Autodesk Fusion 360 part; units mm, degrees
(part 2 of 3)
sketch "Sketch5" plane through (0, 0, 1.5) normal (0, 0, 1) x (-1, 0, 0)
  line L0 (17.5, -111.5) -> (17.5, -101.5)
  line L1 (17.5, -101.5) -> (28.75, -101.5)
  line L2 (28.75, -101.5) -> (28.75, -111.5)
  line L3 (28.75, -111.5) -> (17.5, -111.5)
  arc A0 (29, -9) -> (20, 0) centre (20, -9) ccw
  line L4 (20, 0) -> (-20, 0)
  arc A1 (-20, 0) -> (-29, -9) centre (-20, -9) ccw
  line L5 (-29, -9) -> (-29, -117)
  arc A2 (-29, -117) -> (-20, -126) centre (-20, -117) ccw
  line L6 (-20, -126) -> (20, -126)
  arc A3 (20, -126) -> (29, -117) centre (20, -117) ccw
  line L7 (29, -117) -> (29, -9)
  circle A4 centre (-23.5, -110) radius 1.5
  line L8 (-23.5, -108.5) -> (-27.7, -108.5)
  line L9 (-27.7, -108.5) -> (-27.7, -83)
  line L10 (-27.7, -83) -> (-22.7, -83)
  line L11 (-22.7, -83) -> (-22.7, -108.5)
  line L12 (-22.7, -108.5) -> (-23.5, -108.5)
  circle A5 centre (23.5, -24) radius 1.5
  circle A6 centre (23.5, -116) radius 1.5
  circle A7 centre (-23.5, -30) radius 1.5
  line L13 (-22.7, -58.9) -> (-27.7, -58.9)
  line L14 (-27.7, -58.9) -> (-27.7, -33.4)
  line L15 (-27.7, -33.4) -> (-22.7, -33.4)
  line L16 (-22.7, -33.4) -> (-22.7, -58.9)
  line L17 (27.7, -98) -> (22.7, -98)
  line L18 (22.7, -98) -> (22.7, -77.5)
  line L19 (22.7, -77.5) -> (27.7, -77.5)
  line L20 (27.7, -77.5) -> (27.7, -98)
  line L21 (-22.7, -81.7) -> (-27.7, -81.7)
  line L22 (-27.7, -81.7) -> (-27.7, -61.2)
  line L23 (-27.7, -61.2) -> (-22.7, -61.2)
  line L24 (-22.7, -61.2) -> (-22.7, -81.7)
  line L25 (27.7, -52.4) -> (22.7, -52.4)
  line L26 (22.7, -52.4) -> (22.7, -26.9)
  line L27 (22.7, -26.9) -> (27.7, -26.9)
  line L28 (27.7, -26.9) -> (27.7, -52.4)
  line L29 (27.7, -75.2) -> (22.7, -75.2)
  line L30 (22.7, -75.2) -> (22.7, -54.7)
  line L31 (22.7, -54.7) -> (27.7, -54.7)
  line L32 (27.7, -54.7) -> (27.7, -75.2)
  line L33 (-29, -126) -> (-11, -126)
  line L34 (-11, -126) -> (-18.5, -126)
  line L35 (-11, -126) -> (-11, -127.2)
  line L36 (-11, -127.2) -> (-18.5, -127.2)
  line L37 (-18.5, -127.2) -> (-18.5, -126)
  line L38 (-11, -126) -> (-11, -122)
  line L39 (-11, -122) -> (-18.5, -122)
  line L40 (-18.5, -122) -> (-18.5, -126)
  line L41 (-11, -125) -> (-7.5, -125)
  line L42 (-7.5, -125.5) -> (-7.5, -127.8)
  line L43 (-7.5, -125.5) -> (-5.5, -125.5)
  line L44 (-5.5, -125.5) -> (-5.5, -127.8)
  line L45 (-5.5, -127.8) -> (-7.5, -127.8)
  line L46 (-5.5, -126.65) -> (-5, -126.65) construction
  line L47 (-3, -127.8) -> (-5, -127.8)
  line L48 (-3, -125.5) -> (-3, -127.8)
  line L49 (-5, -125.5) -> (-3, -125.5)
  line L50 (-5, -125.5) -> (-5, -127.8)
  line L51 (-0.5, -127.8) -> (-2.5, -127.8)
  line L52 (-0.5, -125.5) -> (-0.5, -127.8)
  line L53 (-2.5, -125.5) -> (-0.5, -125.5)
  line L54 (-2.5, -125.5) -> (-2.5, -127.8)
  line L55 (2, -127.8) -> (0, -127.8)
  line L56 (0, -125.5) -> (0, -127.8)
  line L57 (2, -125.5) -> (2, -127.8)
  line L58 (0, -125.5) -> (2, -125.5)
  line L59 (2, -127.8) -> (0, -127.8)
  line L60 (2, -125.5) -> (2, -127.8)
  line L61 (0, -125.5) -> (2, -125.5)
  line L62 (0, -125.5) -> (0, -127.8)
  line L63 (-0.5, -125.5) -> (-0.5, -127.8)
  line L64 (-0.5, -127.8) -> (-2.5, -127.8)
  line L65 (-2.5, -125.5) -> (-2.5, -127.8)
  line L66 (-2.5, -125.5) -> (-0.5, -125.5)
  line L67 (-5, -125.5) -> (-3, -125.5)
  line L68 (-3, -125.5) -> (-3, -127.8)
  line L69 (-3, -127.8) -> (-5, -127.8)
  line L70 (-5, -125.5) -> (-5, -127.8)
  line L71 (-5.5, -127.8) -> (-7.5, -127.8)
  line L72 (-5.5, -125.5) -> (-5.5, -127.8)
  line L73 (-7.5, -125.5) -> (-5.5, -125.5)
  line L74 (-7.5, -125.5) -> (-7.5, -127.8)
  line L75 (14.5, -125.5) -> (14.5, -127.8)
  line L76 (14.5, -127.8) -> (12.5, -127.8)
  line L77 (12.5, -125.5) -> (14.5, -125.5)
  line L78 (12.5, -125.5) -> (12.5, -127.8)
  line L79 (12, -125.5) -> (12, -127.8)
  line L80 (12, -127.8) -> (10, -127.8)
  line L81 (10, -125.5) -> (10, -127.8)
  line L82 (10, -125.5) -> (12, -125.5)
  line L83 (9.5, -127.8) -> (7.5, -127.8)
  line L84 (9.5, -125.5) -> (9.5, -127.8)
  line L85 (7.5, -125.5) -> (9.5, -125.5)
  line L86 (7.5, -125.5) -> (7.5, -127.8)
  line L87 (7, -125.5) -> (7, -127.8)
  line L88 (7, -127.8) -> (5, -127.8)
  line L89 (5, -125.5) -> (7, -125.5)
  line L90 (5, -125.5) -> (5, -127.8)
  line L91 (-29, -9) -> (-20.7, -9)
  line L92 (-20.7, -0.0273) -> (-20.7, -7.1273)
  line L93 (-20.7, -7.1273) -> (-13.2, -7.1273)
  line L94 (-13.2, -7.1273) -> (-13.2, 0)
  line L95 (-20.7, -0.0273) -> (-13.2, 0)
  line L96 (-16.95, -0.0136) -> (-16.9558, 1.5864)
  line L97 (-16.95, -0.0136) -> (-16.9573, 1.9864)
  arc A8 (-13.2, 0) -> (-20.7, -0.0273) centre (-16.9369, -3.6082) ccw
  circle A9 centre (-16.9409, -2.5136) radius 4.5
  dimension "d100" = 18
  dimension "d101" = 7.5
  dimension "d102" = 1.2
  dimension "d103" = 4
  dimension "d112" = 3.5
  dimension "d114" = 2.3
  dimension "d115" = 2
  dimension "d116" = 2.3
  dimension "d117" = 0.5
  dimension "d118" = 2.3
  dimension "d119" = 2
  dimension "d120" = 2.3
  dimension "d121" = 2.3
  dimension "d122" = 2
  dimension "d123" = 2.3
  dimension "d124" = 2.3
  dimension "d125" = 2
  dimension "d126" = 2.3
  dimension "d143" = 2.3
  dimension "d144" = 2
  dimension "d145" = 2.3
  dimension "d146" = 2.3
  dimension "d147" = 2
  dimension "d148" = 2.3
  dimension "d149" = 2.3
  dimension "d150" = 2
  dimension "d151" = 2.3
  dimension "d152" = 2.3
  dimension "d153" = 2
  dimension "d154" = 2.3
  dimension "d155" = 2.3
  dimension "d156" = 2
  dimension "d157" = 2.3
  dimension "d158" = 2.3
  dimension "d159" = 2
  dimension "d160" = 2.3
  dimension "d161" = 2.3
  dimension "d162" = 2
  dimension "d163" = 2.3
  dimension "d164" = 2.3
  dimension "d165" = 2
  dimension "d166" = 2.3
  dimension "d169" = 8.3
  dimension "d170" = 7.1
  dimension "d171" = 7.5
  dimension "d172" = 1.6
  dimension "d173" = 2
  dimension "d174" = 9
  constraint perpendicular L5 L33
  constraint parallel L33 L34
  constraint perpendicular L6 L35
  constraint perpendicular L35 L36
  constraint perpendicular L34 L38
  constraint perpendicular L38 L39
  constraint coincident L38 L41.start
  constraint perpendicular L38 L41
  constraint perpendicular L6 L42
  constraint perpendicular L42 L43
  constraint perpendicular L6 L44
  constraint midpoint L44 L46.start
  constraint perpendicular L44 L46
  constraint perpendicular L49 L50
  constraint perpendicular L53 L54
  constraint perpendicular L56 L58
  constraint perpendicular L73 L74
  constraint perpendicular L67 L70
  constraint perpendicular L65 L66
  constraint perpendicular L61 L62
  constraint perpendicular L89 L90
  constraint perpendicular L85 L86
  constraint perpendicular L81 L82
  constraint perpendicular L77 L78
  constraint coincident A1.end L5.start
  constraint perpendicular L5 L91
  constraint coincident A1 L92.start
  constraint perpendicular L91 L92
  constraint perpendicular L92 L93
  constraint coincident L4 L94.end
  constraint perpendicular L4 L94
  constraint midpoint L95 L96.start
  constraint perpendicular L95 L96
  constraint perpendicular L95 L97
  constraint coincident L96.end A8
  constraint coincident L97.end A9
  measures "d100" distance of L33.start L33.end
  measures "d101" distance of L33.end L34.end
  measures "d102" distance of L33.end L35.end
  measures "d103" distance of L33.end L38.end
  measures "d112" distance of L41.start L41.end
  measures "d114" distance of L42.start L42.end
  measures "d115" distance of L42.start L43.end
  measures "d116" distance of L43.end L44.end
  measures "d117" distance of L46.start L46.end
  measures "d118" distance of L49.start L47.end
  measures "d119" distance of L49.start L48.start
  measures "d120" distance of L47.start L48.start
  measures "d121" distance of L53.start L51.end
  measures "d122" distance of L53.start L52.start
  measures "d123" distance of L51.start L52.start
  measures "d124" distance of L55.end L56.start
  measures "d125" distance of L57.start L56.start
  measures "d126" distance of L57.start L55.start
  measures "d143" distance of L42.start L42.end
  measures "d144" distance of L42.start L43.end
  measures "d145" distance of L44.end L43.end
  measures "d146" distance of L49.start L47.end
  measures "d147" distance of L49.start L48.start
  measures "d148" distance of L47.start L48.start
  measures "d149" distance of L51.end L53.start
  measures "d150" distance of L52.start L53.start
  measures "d151" distance of L52.start L51.start
  measures "d152" distance of L55.end L56.start
  measures "d153" distance of L57.start L56.start
  measures "d154" distance of L57.start L55.start
  measures "d155" distance of L89.start L88.end
  measures "d156" distance of L89.start L87.start
  measures "d157" distance of L87.end L87.start
  measures "d158" distance of L85.start L83.end
  measures "d159" distance of L85.start L84.start
  measures "d160" distance of L83.start L84.start
  measures "d161" distance of L80.end L81.start
  measures "d162" distance of L79.start L81.start
  measures "d163" distance of L79.start L79.end
  measures "d164" distance of L76.end L77.start
  measures "d165" distance of L75.start L77.start
  measures "d166" distance of L75.start L75.end
  measures "d169" distance of A1.end L91.end
  measures "d170" distance of L92.start L92.end
  measures "d171" distance of L92.end L93.end
  measures "d172" distance of L96.start L96.end
  measures "d173" distance of L96.start L97.end
  measures "d174" diameter of A9
extrude "Extrude8" add sketch "Sketch5" along normal blind 3 separate body contours L6 L33 L34 L38 L39 L40 | L6 L33 L34 L35 L36 L37 makes body 2
fillet "Fillet2" radius 1 6 edges at (18.5, 124, 1.5) (18.5, 126.6, 1.5) (18.5, 124, 4.5) (18.5, 126.6, 4.5) (11, 124.6, 4.5) (11, 124.6, 1.5) on bodies 2
sketch "Sketch6" plane through (0, 127.2, 0) normal (0, 1, 0) x (-1, 0, 0)
  arc A0 (-12, 1.5) -> (-11, 2.5) centre (-12, 2.5) ccw
  line L0 (-11, 2.5) -> (-11, 3.5)
  arc A1 (-11, 3.5) -> (-12, 4.5) centre (-12, 3.5) ccw
  line L1 (-12, 4.5) -> (-17.5, 4.5)
  arc A2 (-17.5, 4.5) -> (-18.5, 3.5) centre (-17.5, 3.5) ccw
  line L2 (-18.5, 3.5) -> (-18.5, 2.5)
  arc A3 (-18.5, 2.5) -> (-17.5, 1.5) centre (-17.5, 2.5) ccw
  line L3 (-17.5, 1.5) -> (-12, 1.5)
  line L4 (-17, 2) -> (-12.5, 2)
  arc A4 (-12.5, 2) -> (-12.5, 4) centre (-12.5, 3) ccw
  line L5 (-12.5, 4) -> (-17, 4)
  arc A5 (-17, 4) -> (-17, 2) centre (-17, 3) ccw
  line L6 (-17, 3) -> (-12.5, 3) construction
  constraint tangent L4 A4
  constraint tangent A4 L5
  constraint parallel L4 L5
  constraint tangent L5 A5
  constraint tangent L4 A5
  constraint perpendicular L0 L6
extrude "Extrude9" cut sketch "Sketch6" against normal blind 5 contours L4 A4 L5 A5 bodies 2
sketch "Sketch7" plane through (0, 122.2, 0) normal (0, 1, 0) x (-1, 0, 0)
  arc A0 (-17, 4) -> (-17, 2) centre (-17, 3) ccw
  line L0 (-17, 2) -> (-12.5, 2)
  arc A1 (-12.5, 2) -> (-12.5, 4) centre (-12.5, 3) ccw
  line L1 (-12.5, 4) -> (-17, 4)
  line L2 (-17, 3) -> (-12.5, 3)
  line L3 (-12.5, 3) -> (-12.5, 2.5)
  line L4 (-12.5, 2.5) -> (-17, 2.5)
  line L5 (-17, 2.5) -> (-17, 3)
  constraint horizontal L2
  constraint vertical L3
  constraint horizontal L4
  constraint vertical L5
  constraint coincident A0.centre L2.start
extrude "Extrude10" add sketch "Sketch7" along normal blind 4 contours L2 L3 L4 L5 bodies 2
extrude "Extrude11" add sketch "Sketch5" along normal blind 2.3 contours L6 L55 L56 L57 L59 L60 L62 | L6 L56 L57 L58 L60 L61 L62 | L6 L42 L43 L44 L72 L73 L74 | L6 L42 L44 L45 L71 L72 L74 | L6 L51 L52 L54 L63 L64 L65 | L6 L52 L53 L54 L63 L65 L66 | L6 L48 L49 L50 L67 L68 L70 | L6 L47 L48 L50 L68 L69 L70 bodies 1
ref_plane "WorkPlane1" through (-1, 126.65, 2.65) normal (1, 0, 0) x (0, 1, 0)
sketch "Sketch8" plane through (-1, 0, 0) normal (1, 0, 0) x (0, 1, 0)
  line L0 (123.5, 1.5) -> (123.5, 2.1)
  line L1 (124.05, 2.65) -> (125.5, 2.65)
  arc A0 (124.05, 2.65) -> (123.5, 2.1) centre (124.05, 2.1) ccw
  line L2 (127.8, 2.65) -> (133.8, 2.65)
  dimension "d132" = 0.55
  dimension "d137" = 6
  constraint tangent L0 A0
  constraint tangent L1 A0
  constraint parallel L1 L2
  measures "d132" radius of A0
  measures "d137" distance of L2.start L2.end
pipe "Pipe1" add square section size 0.5 path "Sketch8" along L1 A0 L0 separate body makes body 3
copy_body "CopyPasteBodies1" bodies 3 makes body 4
move_body "Move1" bodies 4 to x (1, 0, 0) y (0, 1, 0) z (0, 0, 1) at (2.5, 0, 0)
copy_body "CopyPasteBodies2" bodies 4 makes body 5
move_body "Move2" bodies 5 to x (1, 0, 0) y (0, 1, 0) z (0, 0, 1) at (2.5, 0, 0)
copy_body "CopyPasteBodies3" bodies 5 makes body 6
move_body "Move3" bodies 6 to x (1, 0, 0) y (0, 1, 0) z (0, 0, 1) at (2.5, 0, 0)
pipe "Pipe2" add square section size 0.5 path "Sketch8" along L2 separate body makes body 7
copy_body "CopyPasteBodies4" bodies 7 makes body 8
move_body "Move4" bodies 8 to x (1, 0, 0) y (0, 1, 0) z (0, 0, 1) at (2.5, 0, 0)
copy_body "CopyPasteBodies5" bodies 8 makes body 9
move_body "Move5" bodies 9 to x (1, 0, 0) y (0, 1, 0) z (0, 0, 1) at (2.5, 0, 0)
copy_body "CopyPasteBodies6" bodies 9 makes body 10
move_body "Move6" bodies 10 to x (1, 0, 0) y (0, 1, 0) z (0, 0, 1) at (2.5, 0, 0)
chamfer "Chamfer1" distance 0.15 angle 45 16 edges at (-1, 133.8, 2.9) (-0.75, 133.8, 2.65) (-1, 133.8, 2.4) (-1.25, 133.8, 2.65) (6.5, 133.8, 2.9) (6.75, 133.8, 2.65) (6.25, 133.8, 2.65) (6.5, 133.8, 2.4) (1.5, 133.8, 2.9) (1.75, 133.8, 2.65) (1.25, 133.8, 2.65) (1.5, 133.8, 2.4) (4, 133.8, 2.9) (4.25, 133.8, 2.65) (3.75, 133.8, 2.65) (4, 133.8, 2.4) on bodies 7 8 9 10
extrude "Extrude12" add sketch "Sketch5" along normal blind 2.3 contours L6 L75 L76 L78 | L6 L75 L77 L78 | L6 L79 L80 L81 | L6 L79 L81 L82 | L6 L83 L84 L86 | L6 L84 L85 L86 | L6 L87 L88 L90 | L6 L87 L89 L90 bodies 1
copy_body "CopyPasteBodies7" bodies 3 7 9 6 8 10 4 5 makes body 11 makes body 12 makes body 13 makes body 14 makes body 15 makes body 16 makes body 17 makes body 18
move_body "Move7" bodies 11 12 13 14 15 16 17 18 to x (1, 0, 0) y (0, 1, 0) z (0, 0, 1) at (-12.5, 0, 0)
extrude "Extrude13" add sketch "Sketch5" along normal blind 2 separate body contours L92 L94 L95 A9 | L4 L96 L97 A8 A9 | L4 A1 L96 L97 A8 A9 | L92 L93 L94 A9 makes body 19 at (14.7234, -1.0912, 2.8333) makes body 20 at (16.95, 3.3386, 1.5)
extrude "Extrude14" add sketch "Sketch5" along normal blind 3.8 and the other way blind -2.3 separate body contours L4 L95 L96 L97 | L92 L94 L95 A9 | L4 L96 L97 A8 A9 | L94 A9 | L97 A8 A9 | L4 A1 L95 L96 L97 | L4 A1 L96 L97 A8 A9 | L97 A8 A9 | L92 A9 makes body 21
sketch "Sketch9" plane through (0, 0, 0) normal (0, 0, -1) x (1, 0, 0)
  circle A0 centre (23.5, -110) radius 1.5
  arc A1 (-20, 0) -> (-29, -9) centre (-20, -9) ccw
  line L0 (-29, -9) -> (-29, -117)
  arc A2 (-29, -117) -> (-20, -126) centre (-20, -117) ccw
  line L1 (-20, -126) -> (20, -126)
  arc A3 (20, -126) -> (29, -117) centre (20, -117) ccw
  line L2 (29, -117) -> (29, -9)
  arc A4 (29, -9) -> (20, 0) centre (20, -9) ccw
  line L3 (20, 0) -> (-20, 0)
  circle A5 centre (-23.5, -24) radius 1.5
  circle A6 centre (-23.5, -116) radius 1.5
  circle A7 centre (23.5, -30) radius 1.5
  circle A8 centre (-20, -9) radius 3.85
  circle A9 centre (20, -9) radius 3.85
  circle A10 centre (-15, -105) radius 3.85
  circle A11 centre (15, -105) radius 3.85
  circle A12 centre (-20, -9) radius 3.25
  circle A13 centre (20, -9) radius 3.25
  circle A14 centre (-15, -105) radius 3.25
  circle A15 centre (15, -105) radius 3.25
  dimension "d181" = 7.7
  dimension "d182" = 7.7
  dimension "d183" = 7.7
  dimension "d184" = 7.7
  dimension "d185" = 6.5
  dimension "d186" = 6.5
  dimension "d187" = 6.5
  dimension "d188" = 6.5
  constraint concentric A1 A8
  constraint concentric A4 A9
  constraint concentric A8 A12
  constraint concentric A4 A13
  constraint concentric A10 A14
  constraint concentric A11 A15
  measures "d181" diameter of A8
  measures "d182" diameter of A9
  measures "d183" diameter of A10
  measures "d184" diameter of A11
  measures "d185" diameter of A12
  measures "d186" diameter of A13
  measures "d187" diameter of A14
  measures "d188" diameter of A15
extrude "Extrude15" add sketch "Sketch9" along normal blind 5.4 contours A12 | A13 | A14 | A15 bodies 1
extrude "Extrude16" add sketch "Sketch9" along normal blind 1 contours A8 | A9 | A10 | A11 bodies 1
equation "d62 = 7.2 mm + 1.5 mm"

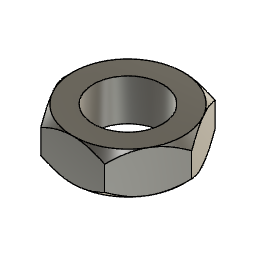
design "5mm Nut"
Autodesk Fusion 360 part; units mm, degrees
sketch "Sketch1" plane through (0, 0, 0) normal (0, 0, 1) x (1, 0, 0)
  circle A0 centre (0, 0) radius 2.5
  circle A1 centre (0, 0) radius 4
  line L0 (-2.3094, 4) -> (-4.6188, 0)
  line L1 (-4.6188, 0) -> (-2.3094, -4)
  line L2 (-2.3094, -4) -> (2.3094, -4)
  line L3 (2.3094, -4) -> (4.6188, 0)
  line L4 (4.6188, 0) -> (2.3094, 4)
  line L5 (2.3094, 4) -> (-2.3094, 4)
  dimension "d1" = 5
  dimension "d2" = 8
  constraint coincident A0.centre A1.centre
  measures "d1" diameter of A0
  measures "d2" diameter of A1
extrude "Extrude1" add sketch "Sketch1" along normal blind 3
sketch "Sketch2" plane through (0, 0, 3) normal (0, 0, 1) x (-1, 0, 0)
  circle A0 centre (0, 0) radius 2.5
  line L0 (-2.3094, -4) -> (2.3094, -4)
  line L1 (2.3094, -4) -> (4.6188, 0)
  line L2 (4.6188, 0) -> (2.3094, 4)
  line L3 (2.3094, 4) -> (-2.3094, 4)
  line L4 (-2.3094, 4) -> (-4.6188, 0)
  line L5 (-4.6188, 0) -> (-2.3094, -4)
  circle A1 centre (0, 0) radius 4
  constraint coincident A0.centre A1.centre
  constraint tangent L0 A1
extrude "Extrude2" cut sketch "Sketch2" against normal blind 6 draft 45 contours A1 keep common part
sketch "Sketch3" plane through (0, 0, 0) normal (0, 0, -1) x (1, 0, 0)
  circle A0 centre (0, 0) radius 2.5
  line L0 (-2.3094, -4) -> (2.3094, -4)
  line L1 (2.3094, -4) -> (4.6188, 0)
  line L2 (4.6188, 0) -> (2.3094, 4)
  line L3 (2.3094, 4) -> (-2.3094, 4)
  line L4 (-2.3094, 4) -> (-4.6188, 0)
  line L5 (-4.6188, 0) -> (-2.3094, -4)
  circle A1 centre (0, 0) radius 4
  constraint concentric A0 A1
  constraint tangent L3 A1
extrude "Extrude3" cut sketch "Sketch3" against normal blind 9 draft 45 contours A1 keep common part

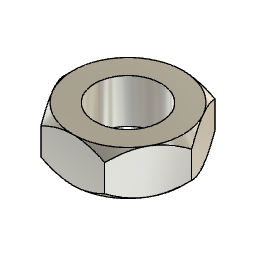
design "3mm_Nut"
Autodesk Fusion 360 part; units mm, degrees
sketch "Sketch1" plane through (0, 0, 0) normal (0, 0, 1) x (1, 0, 0)
  circle A0 centre (0, 0) radius 1.5
  line L0 (-1.4434, 2.5) -> (-2.8868, 0)
  line L1 (-2.8868, 0) -> (-1.4434, -2.5)
  line L2 (-1.4434, -2.5) -> (1.4434, -2.5)
  line L3 (1.4434, -2.5) -> (2.8868, 0)
  line L4 (2.8868, 0) -> (1.4434, 2.5)
  line L5 (1.4434, 2.5) -> (-1.4434, 2.5)
  dimension "d1" = 3
  constraint coincident A0.centre origin
  measures "d1" diameter of A0
extrude "Extrude1" add sketch "Sketch1" along normal blind 2
sketch "Sketch2" plane through (0, 0, 2) normal (0, 0, 1) x (-1, 0, 0)
  circle A0 centre (0, 0) radius 1.5
  line L0 (-1.4434, -2.5) -> (1.4434, -2.5)
  line L1 (1.4434, -2.5) -> (2.8868, 0)
  line L2 (2.8868, 0) -> (1.4434, 2.5)
  line L3 (1.4434, 2.5) -> (-1.4434, 2.5)
  line L4 (-1.4434, 2.5) -> (-2.8868, 0)
  line L5 (-2.8868, 0) -> (-1.4434, -2.5)
  circle A1 centre (0, 0) radius 2.5
  constraint coincident A0.centre A1.centre
  constraint tangent L0 A1
extrude "Extrude2" cut sketch "Sketch2" against normal blind 7 draft 45 contours A1 keep common part
sketch "Sketch3" plane through (0, 0, 0) normal (0, 0, -1) x (1, 0, 0)
  circle A0 centre (0, 0) radius 1.5
  line L0 (-1.4434, -2.5) -> (1.4434, -2.5)
  line L1 (1.4434, -2.5) -> (2.8868, 0)
  line L2 (2.8868, 0) -> (1.4434, 2.5)
  line L3 (1.4434, 2.5) -> (-1.4434, 2.5)
  line L4 (-1.4434, 2.5) -> (-2.8868, 0)
  line L5 (-2.8868, 0) -> (-1.4434, -2.5)
  circle A1 centre (0, 0) radius 2.5
  constraint concentric A0 A1
  constraint tangent L0 A1
extrude "Extrude3" cut sketch "Sketch3" against normal blind 5 draft 45 contours A1 keep common part

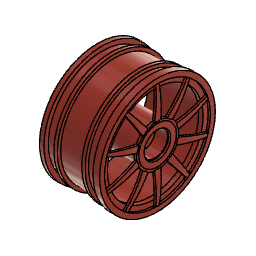
design "Wheel2"
Autodesk Fusion 360 part; units mm, degrees
sketch "Sketch1" plane through (0, 0, 0) normal (0, 1, 0) x (1, 0, 0)
  line L0 (0, -26) -> (-2, -26)
  line L1 (-2, -26) -> (-2, -24)
  line L2 (-2, -24) -> (-6, -24)
  line L3 (-6, -24) -> (-6, -25.5)
  line L4 (-6, -25.5) -> (-7.5, -25.5)
  line L5 (-7.5, -25.5) -> (-7.5, -24)
  line L6 (-7.5, -24) -> (-18.5, -24)
  line L7 (-13, -24) -> (-13, -27.5) construction
  line L8 (-18.5, -25.5) -> (-18.5, -24)
  line L9 (-20, -25.5) -> (-18.5, -25.5)
  line L10 (-20, -24) -> (-20, -25.5)
  line L11 (-24, -24) -> (-20, -24)
  line L12 (-24, -26) -> (-24, -24)
  line L13 (-26, -26) -> (-24, -26)
  line L14 (-13, -24) -> (-13, -27.5) construction
  line L15 (-26, -26) -> (-26, -13)
  line L16 (0, -26) -> (0, -13)
  line L17 (-33, -13) -> (4.5762, -13) construction
  line L18 (0, 0) -> (0, -13)
  line L19 (0, 0) -> (-2, 0)
  line L20 (-2, 0) -> (-2, -2)
  line L21 (-2, -2) -> (-6, -2)
  line L22 (-6, -2) -> (-6, -0.5)
  line L23 (-6, -0.5) -> (-7.5, -0.5)
  line L24 (-7.5, -0.5) -> (-7.5, -2)
  line L25 (-7.5, -2) -> (-18.5, -2)
  line L26 (-18.5, -0.5) -> (-18.5, -2)
  line L27 (-20, -0.5) -> (-18.5, -0.5)
  line L28 (-20, -2) -> (-20, -0.5)
  line L29 (-24, -2) -> (-20, -2)
  line L30 (-24, 0) -> (-24, -2)
  line L31 (-26, 0) -> (-24, 0)
  line L32 (-26, 0) -> (-26, -13)
  line L33 (-26, 0) -> (-26, -3)
  line L34 (-26, -3) -> (-2, -3)
  line L35 (-2, -3) -> (-2, -4.5)
  line L36 (-2, -4.5) -> (0, -4.5)
  dimension "d2" = 26
  dimension "d3" = 2
  dimension "d4" = 2
  dimension "d5" = 4
  dimension "d6" = 1.5
  dimension "d7" = 1.5
  dimension "d8" = 1.5
  dimension "d9" = 11
  dimension "d10" = 13
  dimension "d11" = 13
  dimension "d12" = 3
  dimension "d13" = 1.5
  constraint perpendicular L0 L1
  constraint perpendicular L1 L2
  constraint perpendicular L2 L3
  constraint perpendicular L3 L4
  constraint perpendicular L4 L5
  constraint perpendicular L5 L6
  constraint midpoint L6 L7.start
  constraint perpendicular L6 L7
  constraint symmetric L0.start L7 L13.start
  constraint symmetric L0.end L7 L12.start
  constraint symmetric L1.end L7 L11.start
  constraint symmetric L2.end L7 L10.start
  constraint symmetric L3.end L7 L9.start
  constraint symmetric L4.end L7 L8.start
  constraint symmetric L5.end L7 L6.end
  constraint symmetric L14.start L7 L7.start
  constraint symmetric L14.end L7 L7.end
  constraint perpendicular L13 L15
  constraint perpendicular L0 L16
  constraint perpendicular L16 L17
  constraint symmetric L0.start L17 L18.start
  constraint symmetric L0.end L17 L19.end
  constraint symmetric L1.end L17 L20.end
  constraint symmetric L2.end L17 L21.end
  constraint symmetric L3.end L17 L22.end
  constraint symmetric L4.end L17 L23.end
  constraint symmetric L5.end L17 L24.end
  constraint symmetric L6.end L17 L25.end
  constraint symmetric L8.start L17 L26.start
  constraint symmetric L9.start L17 L27.start
  constraint symmetric L10.start L17 L28.start
  constraint symmetric L11.start L17 L29.start
  constraint symmetric L12.start L17 L30.start
  constraint symmetric L13.start L17 L31.start
  constraint symmetric L15.end L17 L32.end
  constraint symmetric L16.end L17 L18.end
  constraint perpendicular L31 L33
  constraint perpendicular L33 L34
  constraint perpendicular L34 L35
  constraint coincident L18 L36.end
  constraint perpendicular L18 L36
  measures "d2" distance of L18.start L0.start
  measures "d3" distance of L0.start L0.end
  measures "d4" distance of L0.end L1.end
  measures "d5" distance of L1.end L2.end
  measures "d6" distance of L2.end L3.end
  measures "d7" distance of L3.end L4.end
  measures "d8" distance of L4.end L5.end
  measures "d9" distance of L5.end L6.end
  measures "d10" distance of L13.start L15.end
  measures "d11" distance of L0.start L16.end
  measures "d12" distance of L31.start L33.end
  measures "d13" distance of L34.end L35.end
revolve "Revolve1" add sketch "Sketch1" angle 360 about axis through (0, 0, 26) along (-1, 0, 0) contours L18 L19 L20 L21 L22 L23 L24 L25 L26 L27 L28 L29 L30 L31 L32 L33 L34 L35 L36 makes body 1
ref_plane "WorkPlane1" through (0, 0, 26) normal (1, 0, 0) x (0, 0, -1)
sketch "Sketch2" plane through (0, 0, 0) normal (1, 0, 0) x (0, 1, 0)
  circle A0 centre (0, 26) radius 21.5
  circle A1 centre (0, 26) radius 5.5
  circle A2 centre (0, 26) radius 8.5
  circle A3 centre (0, 26) radius 6
  dimension "d16" = 11
  dimension "d17" = 17
  dimension "d18" = 12
  constraint concentric A0 A1
  constraint concentric A0 A2
  constraint concentric A2 A3
  measures "d16" diameter of A1
  measures "d17" diameter of A2
  measures "d18" diameter of A3
extrude "Extrude1" add sketch "Sketch2" along normal blind 1 separate body contours A2 makes body 2
sketch "Sketch3" plane through (0, 0, 0) normal (1, 0, 0) x (0, 1, 0)
  circle A0 centre (0, 26) radius 26
  circle A1 centre (0, 26) radius 21.5
  circle A2 centre (0, 26) radius 23.75
  dimension "d21" = 47.5
  constraint concentric A0 A2
  measures "d21" diameter of A2
extrude "Extrude2" add sketch "Sketch3" along normal blind 1 contours A0 bodies 1
extrude "Extrude3" add sketch "Sketch2" against normal blind 5.5 separate body contours A3 makes body 3
extrude "Extrude4" add sketch "Sketch2" against normal blind 16 contours A2 bodies 2 3
extrude "Extrude5" add sketch "Sketch2" along normal blind -6 and the other way blind 5.5 separate body contours A1 makes body 4
sketch "Sketch4" plane through (0, 0, 0) normal (1, 0, 0) x (0, 1, 0)
  circle A0 centre (0, 26) radius 1.5
  dimension "d32" = 3
  measures "d32" diameter of A0
extrude "Extrude6" cut sketch "Sketch4" against normal blind 30 bodies 4
sketch "Sketch5" plane through (-6, 0, 0) normal (-1, 0, 0) x (0, -1, 0)
  circle A0 centre (0, 26) radius 1.5
  circle A1 centre (0, 26) radius 5.5
  line L0 (-3.4641, 32) -> (-6.9282, 26)
  line L1 (-6.9282, 26) -> (-3.4641, 20)
  line L2 (-3.4641, 20) -> (3.4641, 20)
  line L3 (3.4641, 20) -> (6.9282, 26)
  line L4 (6.9282, 26) -> (3.4641, 32)
  line L5 (3.4641, 32) -> (-3.4641, 32)
  point P0 (0, 26)
  dimension "d35" = 12
  constraint coincident P0 A0.centre
  measures "d35" vertical distance of L0.start L2.end
extrude "Extrude7" cut sketch "Sketch5" along normal blind 47 contours L0 L1 L2 L3 L4 L5 bodies 2
ref_plane "WorkPlane3" through (-2.2433, 0, 26) normal (0, -1, 0) x (0, 0, 1)
sketch "Sketch6" plane through (0, 0, 0) normal (0, -1, 0) x (-1, 0, 0)
  arc A0 (-1, -34.5) -> (-1, -49.75) centre (55, -42.125) ccw
  arc A1 (-0.0254, -34.4777) -> (-0.0556, -49.7496) centre (55.4716, -42.2236) ccw
  line L0 (-1, -34.5) -> (-0.9617, -34.2189)
  line L1 (-0.9617, -34.2189) -> (0.0019, -34.3501)
  line L2 (-0.0254, -34.4777) -> (0.0019, -34.3501)
  line L3 (-0.0556, -49.7496) -> (-1, -49.75)
  constraint tangent A0 A1
  constraint tangent A0 L0
  constraint perpendicular L0 L1
extrude "Extrude8" add sketch "Sketch6" along normal blind 1.5 and the other way blind 1.5 bodies 1 4 2
ref_plane "WorkPlane4" through (1.5167, 0.4718, 42.125) normal (1, 0, 0) x (0, 0, -1)
sketch "Sketch7" plane through (1.5167, 0, 0) normal (1, 0, 0) x (0, 1, 0)
  line L0 (1.5, 49.75) -> (0.0073, 49.75)
  arc A0 (0.0073, 49.75) -> (-0.0073, 49.75) centre (0, 26) ccw
  line L1 (-0.0073, 49.75) -> (-1.5, 49.75)
  line L2 (-1.5, 49.75) -> (-1.5, 34.5)
  line L3 (-1.5, 34.5) -> (0, 34.5)
  line L4 (0, 34.5) -> (1.5, 34.5)
  line L5 (1.5, 34.5) -> (1.5, 49.75)
  line L6 (-0.7536, 49.75) -> (-1.5, 34.365)
  line L7 (-1.5, 34.365) -> (0, 34.5)
  line L8 (0, 34.5) -> (1.4987, 34.365)
  line L9 (1.4987, 34.365) -> (0.7536, 49.75)
  line L10 (0.7536, 49.75) -> (-0.7536, 49.75)
  constraint midpoint L1 L6.start
  constraint coincident L3.end L4.start
  constraint midpoint L0 L9.end
extrude "Extrude9" cut sketch "Sketch7" against normal blind 1.5 contours L0 L4 L5 L9 | L1 L2 L3 L6 bodies 1
pattern_circular "C-Pattern1" count 10 over 360 about axis through (1, 0, 26) along (1, 0, 0) of "Extrude8", "Extrude9"
sketch "Sketch8" plane through (1, 0, 0) normal (1, 0, 0) x (0, 1, 0)
  circle A0 centre (0, 26) radius 6
  arc A1 (0, 34.5) -> (-4.9962, 32.8766) centre (0, 26) ccw
  arc A2 (-4.9962, 32.8766) -> (-8.084, 28.6266) centre (0, 26) ccw
  arc A3 (-8.084, 28.6266) -> (-8.084, 23.3734) centre (0, 26) ccw
  arc A4 (-8.084, 23.3734) -> (-4.9962, 19.1234) centre (0, 26) ccw
  arc A5 (-4.9962, 19.1234) -> (0, 17.5) centre (0, 26) ccw
  arc A6 (0, 17.5) -> (4.9962, 19.1234) centre (0, 26) ccw
  arc A7 (4.9962, 19.1234) -> (8.084, 23.3734) centre (0, 26) ccw
  arc A8 (8.084, 23.3734) -> (8.084, 28.6266) centre (0, 26) ccw
  arc A9 (8.084, 28.6266) -> (4.9962, 32.8766) centre (0, 26) ccw
  arc A10 (4.9962, 32.8766) -> (0, 34.5) centre (0, 26) ccw
  circle A11 centre (0, 26) radius 9.5
  dimension "d49" = 19
  constraint concentric A0 A11
  measures "d49" diameter of A11
extrude "Extrude10" add sketch "Sketch8" along normal blind -1 and the other way blind -0.1 contours A11 bodies 1

design "Pixy2"
Autodesk Fusion 360 part; units mm, degrees
sketch "Sketch1" plane through (0, 0, 0) normal (1, 0, 0) x (0, 1, 0)
  line L0 (0, 0) -> (0, 47.7) construction
  line L1 (-8.85, 0) -> (8.85, 0)
  line L2 (-8.85, 0) -> (-8.85, 4.5)
  line L3 (8.85, 0) -> (8.85, 4.5)
  line L4 (10.85, 6.5) -> (18.85, 6.5)
  line L5 (-10.85, 6.5) -> (-18.85, 6.5)
  line L6 (-18.85, 6.5) -> (-18.85, 42)
  line L7 (18.85, 6.5) -> (18.85, 42)
  line L8 (-18.85, 42) -> (-8.85, 42)
  line L9 (-8.85, 42) -> (-8.85, 43.8)
  line L10 (18.85, 42) -> (8.85, 42)
  line L11 (8.85, 42) -> (8.85, 43.8)
  line L12 (-2.5, 47.7) -> (2.5, 47.7)
  line L13 (-8.85, 43.8) -> (-2.5, 47.7)
  line L14 (8.85, 43.8) -> (2.5, 47.7)
  line L15 (-8.85, 4.5) -> (-10.85, 6.5)
  line L16 (8.85, 4.5) -> (10.85, 6.5)
  point P0 (-8.85, 6.5)
  point P1 (8.85, 6.5)
  dimension "d1" = 47.7
  dimension "d2" = 17.7
  dimension "d5" = 10
  dimension "d6" = 10
  dimension "d7" = 35.5
  dimension "d8" = 35.5
  dimension "d9" = 10
  dimension "d10" = 1.8
  dimension "d11" = 10
  dimension "d12" = 1.8
  dimension "d13" = 5
  dimension "d15" = 2
  dimension "d16" = 2
  dimension "d17" = 2
  dimension "d18" = 2
  constraint coincident L0.start origin
  constraint vertical L0
  constraint horizontal L1
  constraint midpoint L0.start L1
  constraint perpendicular L1 L2
  constraint perpendicular L1 L3
  constraint perpendicular L3 L4
  constraint perpendicular L2 L5
  constraint perpendicular L5 L6
  constraint perpendicular L4 L7
  constraint perpendicular L6 L8
  constraint perpendicular L8 L9
  constraint perpendicular L7 L10
  constraint perpendicular L10 L11
  constraint horizontal L12
  constraint midpoint L0.end L12
  constraint coincident P0 L2
  constraint coincident P0 L5
  constraint coincident P1 L3
  constraint coincident P1 L4
  measures "d1" distance of L0.start L0.end
  measures "d2" distance of L1.start L1.end
  measures "d5" distance of P1 L4.end
  measures "d6" distance of P0 L5.end
  measures "d7" distance of L5.end L6.end
  measures "d8" distance of L4.end L7.end
  measures "d9" distance of L6.end L8.end
  measures "d10" distance of L8.end L9.end
  measures "d11" distance of L7.end L10.end
  measures "d12" distance of L10.end L11.end
  measures "d13" distance of L12.start L12.end
  measures "d15" distance of P0 L2.end
  measures "d16" distance of P0 L5.start
  measures "d17" distance of P1 L3.end
  measures "d18" distance of P1 L4.start
extrude "Extrude1" add sketch "Sketch1" along normal blind 1.5
sketch "Sketch2" plane through (0, 0, 0) normal (-1, 0, 0) x (0, -1, 0)
  line L0 (-8.85, 0) -> (8.85, 0)
  line L1 (8.85, 0) -> (8.85, 4.5)
  line L2 (8.85, 4.5) -> (10.85, 6.5)
  line L3 (10.85, 6.5) -> (18.85, 6.5)
  line L4 (18.85, 6.5) -> (18.85, 42)
  line L5 (18.85, 42) -> (8.85, 42)
  line L6 (8.85, 42) -> (8.85, 43.8)
  line L7 (8.85, 43.8) -> (2.5, 47.7)
  line L8 (2.5, 47.7) -> (-2.5, 47.7)
  line L9 (-2.5, 47.7) -> (-8.85, 43.8)
  line L10 (-8.85, 43.8) -> (-8.85, 42)
  line L11 (-8.85, 42) -> (-18.85, 42)
  line L12 (-18.85, 42) -> (-18.85, 6.5)
  line L13 (-18.85, 6.5) -> (-10.85, 6.5)
  line L14 (-10.85, 6.5) -> (-8.85, 4.5)
  line L15 (-8.85, 4.5) -> (-8.85, 0)
  line L16 (8.85, 43.8) -> (7.35, 43.8)
  line L17 (-8.85, 43.8) -> (-7.35, 43.8)
  line L18 (-7.35, 43.8) -> (7.35, 43.8)
  line L19 (-7.35, 43.8) -> (-7.35, 29.1)
  line L20 (8.1, 43.8) -> (8.1, 29.1)
  line L21 (-7.35, 29.1) -> (8.1, 29.1)
  line L22 (-2.15, 43.8) -> (2.15, 43.8)
  line L23 (-2.15, 43.8) -> (-2.15, 45.35)
  line L24 (2.15, 43.8) -> (2.15, 45.35)
  arc A0 (0, 47.5) -> (-2.15, 45.35) centre (0, 45.35) ccw
  arc A1 (2.15, 45.35) -> (0, 47.5) centre (0, 45.35) ccw
  line L25 (-25.85, 36.45) -> (11.15, 36.45) construction
  line L26 (-25.85, 36.45) -> (11.15, 36.45) construction
  arc A2 (0, 25.4) -> (2.15, 27.55) centre (0, 27.55) ccw
  line L27 (-2.15, 29.1) -> (-2.15, 27.55)
  arc A3 (-2.15, 27.55) -> (0, 25.4) centre (0, 27.55) ccw
  line L28 (2.15, 29.1) -> (2.15, 27.55)
  circle A4 centre (0, 45.35) radius 0.75
  circle A5 centre (0, 27.55) radius 0.75
  point P0 (-2.15, 47.5)
  point P1 (2.15, 47.5)
  dimension "d21" = 1.5
  dimension "d22" = 1.5
  dimension "d23" = 14.7
  dimension "d24" = 14.7
  dimension "d25" = 4.3
  dimension "d26" = 3.7
  dimension "d27" = 3.7
  dimension "d28" = 2.15
  dimension "d29" = 1.5
  dimension "d30" = 1.5
  constraint coincident L6.end L7.start
  constraint perpendicular L6 L16
  constraint coincident L9.end L10.start
  constraint perpendicular L10 L17
  constraint perpendicular L17 L19
  constraint midpoint L16 L20.start
  constraint perpendicular L16 L20
  constraint horizontal L22
  constraint midpoint L18 L22
  constraint perpendicular L22 L23
  constraint perpendicular L22 L24
  constraint coincident P0 L23
  constraint tangent L23 A0
  constraint coincident P1 L24
  constraint tangent L24 A1
  constraint equal A0 A1
  constraint coincident A0.start A1.end
  constraint horizontal L25
  constraint midpoint L19 L25
  constraint symmetric L22.start L25 L27.start
  constraint symmetric L22.end L25 L28.start
  constraint symmetric L23.end L25 L27.end
  constraint symmetric A0.start L25 A2.start
  constraint symmetric A0 L25 A3
  constraint symmetric L24.end L25 A2.end
  constraint symmetric A1 L25 A2
  constraint symmetric L26.start L25 L25.start
  constraint symmetric L26.end L25 L25.end
  constraint concentric A0 A4
  constraint concentric A3 A5
  measures "d21" distance of L6.end L16.end
  measures "d22" distance of L9.end L17.end
  measures "d23" distance of L17.end L19.end
  measures "d24" distance of L20.start L20.end
  measures "d25" distance of L22.start L22.end
  measures "d26" distance of L22.start P0
  measures "d27" distance of L22.end P1
  measures "d28" radius of A0
  measures "d29" diameter of A4
  measures "d30" diameter of A5
extrude "Extrude2" add sketch "Sketch2" along normal blind 4.2 contours L16 L18 L19 L20 L21 L22 | L18 L22 L23 L24 A0 A1 | L21 A2 L27 A3 L28
sketch "Sketch3" plane through (-4.2, 0, 0) normal (-1, 0, 0) x (0, -1, 0)
  circle A0 centre (0, 27.55) radius 0.75
  circle A1 centre (0, 45.35) radius 0.75
  line L0 (8.1, 43.8) -> (2.15, 43.8)
  line L1 (2.15, 43.8) -> (2.15, 45.35)
  arc A2 (2.15, 45.35) -> (-2.15, 45.35) centre (0, 45.35) ccw
  line L2 (-2.15, 45.35) -> (-2.15, 43.8)
  line L3 (-2.15, 43.8) -> (-7.35, 43.8)
  line L4 (-7.35, 43.8) -> (-7.35, 29.1)
  line L5 (-7.35, 29.1) -> (-2.15, 29.1)
  line L6 (-2.15, 29.1) -> (-2.15, 27.55)
  arc A3 (-2.15, 27.55) -> (2.15, 27.55) centre (0, 27.55) ccw
  line L7 (2.15, 27.55) -> (2.15, 29.1)
  line L8 (2.15, 29.1) -> (8.1, 29.1)
  line L9 (8.1, 29.1) -> (8.1, 43.8)
  line L10 (-7.35, 36.45) -> (8.1, 36.45) construction
  line L11 (0, 47.5) -> (0, 25.4) construction
  circle A4 centre (0, 36.45) radius 6.7
  dimension "d33" = 13.4
  constraint midpoint L4 L10.start
  constraint midpoint L9 L10.end
  constraint midpoint A2 L11.start
  constraint midpoint A3 L11.end
  constraint midpoint L11 A4.centre
  measures "d33" diameter of A4
extrude "Extrude3" add sketch "Sketch3" along normal blind 6.2 contours A4
sketch "Sketch4" plane through (0, -8.1, 0) normal (0, -1, 0) x (1, 0, 0)
  line L0 (0, 29.1) -> (0, 43.8)
  line L1 (0, 43.8) -> (-4.2, 43.8)
  line L2 (-4.2, 43.8) -> (-4.2, 29.1)
  line L3 (-4.2, 29.1) -> (0, 29.1)
  line L4 (-10.4, 43.15) -> (-10.4, 29.75)
  line L5 (-4.2, 29.75) -> (-4.2, 43.15)
  line L6 (-10.4, 43.15) -> (-6.7, 43.15)
  line L7 (-10.4, 29.75) -> (-6.7, 29.75)
  line L8 (-10.4, 43.15) -> (-5.4, 43.15)
  line L9 (-10.4, 29.75) -> (-5.4, 29.75)
  line L10 (-5.4, 43.15) -> (-5.4, 29.75)
  line L11 (-6.7, 43.15) -> (-6.7, 29.75)
  dimension "d36" = 3.7
  dimension "d37" = 3.7
  dimension "d38" = 5
  dimension "d39" = 5
  constraint coincident L4.start L6.start
  constraint perpendicular L4 L6
  constraint coincident L4.end L7.start
  constraint perpendicular L4 L7
  constraint perpendicular L4 L8
  constraint perpendicular L4 L9
  measures "d36" distance of L4.start L6.end
  measures "d37" distance of L4.end L7.end
  measures "d38" distance of L4.start L8.end
  measures "d39" distance of L4.end L9.end
ref_plane "WorkPlane1" through (-5.4, 0, 36.45) normal (-1, 0, 0) x (0, -1, 0)
sketch "Sketch5" plane through (-5.4, 0, 0) normal (-1, 0, 0) x (0, -1, 0)
  circle A0 centre (0, 36.45) radius 6.7
  circle A1 centre (0, 36.45) radius 6.7
  circle A2 centre (0, 36.45) radius 5.5
  dimension "d41" = 11
  constraint concentric A0 A1
  constraint concentric A1 A2
  measures "d41" diameter of A2
extrude "Extrude4" cut sketch "Sketch5" along normal blind 1.3
sketch "Sketch6" plane through (-10.4, 0, 0) normal (-1, 0, 0) x (0, -1, 0)
  circle A0 centre (0, 36.45) radius 6.7
  circle A1 centre (0, 36.45) radius 3.5
  circle A2 centre (0, 36.45) radius 1.25
  dimension "d44" = 7
  dimension "d45" = 2.5
  constraint concentric A0 A1
  constraint concentric A0 A2
  measures "d44" diameter of A1
  measures "d45" diameter of A2
extrude "Extrude5" add sketch "Sketch6" along normal blind 0.1 contours A1
sketch "Sketch7" plane through (1.5, 0, 0) normal (1, 0, 0) x (0, 1, 0)
  line L0 (-8.85, 0) -> (8.85, 0)
  line L1 (8.85, 0) -> (8.85, 4.5)
  line L2 (8.85, 4.5) -> (10.85, 6.5)
  line L3 (10.85, 6.5) -> (18.85, 6.5)
  line L4 (18.85, 6.5) -> (18.85, 42)
  line L5 (18.85, 42) -> (8.85, 42)
  line L6 (8.85, 42) -> (8.85, 43.8)
  line L7 (8.85, 43.8) -> (2.5, 47.7)
  line L8 (2.5, 47.7) -> (-2.5, 47.7)
  line L9 (-2.5, 47.7) -> (-8.85, 43.8)
  line L10 (-8.85, 43.8) -> (-8.85, 42)
  line L11 (-8.85, 42) -> (-18.85, 42)
  line L12 (-18.85, 42) -> (-18.85, 6.5)
  line L13 (-18.85, 6.5) -> (-10.85, 6.5)
  line L14 (-10.85, 6.5) -> (-8.85, 4.5)
  line L15 (-8.85, 4.5) -> (-8.85, 0)
  line L16 (-4.85, 0) -> (4.85, 0)
  line L17 (4.85, 0) -> (4.85, 3.5) construction
  line L18 (-4.85, 0) -> (-4.85, 3.5) construction
  circle A0 centre (-3.35, 3.5) radius 1.5
  circle A1 centre (3.35, 3.5) radius 1.5
  line L19 (15.35, 6.5) -> (15.35, 9) construction
  circle A2 centre (15.35, 10.5) radius 1.5
  line L20 (13.6, 13.4) -> (13.6, 20.9) construction
  line L21 (11.1, 13.4) -> (16.1, 13.4)
  line L22 (11.1, 13.4) -> (11.1, 20.9)
  line L23 (11.1, 20.9) -> (16.1, 20.9)
  line L24 (16.1, 20.9) -> (16.1, 13.4)
  line L25 (12.5002, 19.75) -> (11.9998, 19.75)
  line L26 (11.9998, 19.75) -> (11.9998, 20.25)
  line L27 (11.9998, 20.25) -> (12.5002, 20.25)
  line L28 (12.5002, 20.25) -> (12.5002, 19.75)
  line L29 (12.5002, 19.75) -> (11.9998, 20.25) construction
  line L30 (11.9998, 19.75) -> (12.5002, 20.25) construction
  line L31 (14.6998, 20.25) -> (15.2002, 20.25)
  line L32 (14.6998, 19.75) -> (14.6998, 20.25)
  line L33 (15.2002, 20.25) -> (15.2002, 19.75)
  line L34 (15.2002, 19.75) -> (14.6998, 19.75)
  line L35 (11.9998, 17.5) -> (12.5002, 17.5)
  line L36 (11.9998, 17) -> (11.9998, 17.5)
  line L37 (12.5002, 17.5) -> (12.5002, 17)
  line L38 (12.5002, 17) -> (11.9998, 17)
  line L39 (14.6998, 17.5) -> (15.2002, 17.5)
  line L40 (14.6998, 17) -> (14.6998, 17.5)
  line L41 (15.2002, 17.5) -> (15.2002, 17)
  line L42 (15.2002, 17) -> (14.6998, 17)
  line L43 (11.9998, 14.75) -> (12.5002, 14.75)
  line L44 (11.9998, 14.25) -> (11.9998, 14.75)
  line L45 (12.5002, 14.75) -> (12.5002, 14.25)
  line L46 (12.5002, 14.25) -> (11.9998, 14.25)
  line L47 (14.6998, 14.75) -> (15.2002, 14.75)
  line L48 (14.6998, 14.25) -> (14.6998, 14.75)
  line L49 (15.2002, 14.75) -> (15.2002, 14.25)
  line L50 (15.2002, 14.25) -> (14.6998, 14.25)
  point P0 (12.25, 20)
  dimension "d48" = 9.7
  dimension "d49" = 3.5
  dimension "d50" = 3.5
  dimension "d53" = 3
  dimension "d54" = 3
  dimension "d56" = 2.5
  dimension "d58" = 3
  dimension "d60" = 7.5
  dimension "d61" = 5
  dimension "d62" = 0.5
  dimension "d65" = 2.7
  dimension "d66" = -5.5
  constraint perpendicular L15 L16
  constraint midpoint L0 L16
  constraint perpendicular L0 L17
  constraint perpendicular L16 L18
  constraint coincident L18.end A0
  constraint coincident L17.end A1
  constraint coincident L3 L19.start
  constraint perpendicular L3 L19
  constraint coincident L19.end A2
  constraint horizontal L21
  constraint midpoint L20.start L21
  constraint perpendicular L21 L22
  constraint perpendicular L20 L23
  constraint perpendicular L21 L24
  constraint horizontal L25
  constraint perpendicular L25 L26
  constraint parallel L25 L27
  constraint parallel L26 L28
  constraint coincident L29 P0
  constraint coincident L30 P0
  measures "d48" distance of L16.start L16.end
  measures "d49" distance of L16.end L17.end
  measures "d50" distance of L16.start L18.end
  measures "d53" diameter of A0
  measures "d54" diameter of A1
  measures "d56" distance of L19.start L19.end
  measures "d58" diameter of A2
  measures "d60" distance of L20.start L20.end
  measures "d61" distance of L21.start L21.end
  measures "d62" distance of L25.end L26.end
extrude "Extrude6" add sketch "Sketch7" along normal blind 9 contours L25 L26 L27 L28 | L31 L32 L33 L34 | L35 L36 L37 L38 | L39 L40 L41 L42 | L43 L44 L45 L46 | L47 L48 L49 L50
extrude "Extrude7" add sketch "Sketch7" along normal blind 3 contours L21 L22 L23 L24
chamfer "Chamfer1" distance 0.2 angle 45 6 faces at (10.5, 12.3334, 19.9167) (10.5, 14.8666, 20.0833) (10.5, 14.8666, 17.3333) (10.5, 12.1666, 17.3333) (10.5, 12.1666, 14.5833) (10.5, 14.8666, 14.5833)
sketch "Sketch8" plane through (1.5, 0, 0) normal (1, 0, 0) x (0, 1, 0)
  line L0 (11.1, 13.4) -> (11.1, 20.9)
  line L1 (11.1, 20.9) -> (16.1, 20.9)
  line L2 (16.1, 20.9) -> (16.1, 13.4)
  line L3 (16.1, 13.4) -> (11.1, 13.4)
  line L4 (-8.85, 0) -> (8.85, 0)
  line L5 (8.85, 0) -> (8.85, 4.5)
  line L6 (8.85, 4.5) -> (10.85, 6.5)
  line L7 (10.85, 6.5) -> (18.85, 6.5)
  line L8 (18.85, 6.5) -> (18.85, 42)
  line L9 (18.85, 42) -> (8.85, 42)
  line L10 (8.85, 42) -> (8.85, 43.8)
  line L11 (8.85, 43.8) -> (2.5, 47.7)
  line L12 (2.5, 47.7) -> (-2.5, 47.7)
  line L13 (-2.5, 47.7) -> (-8.85, 43.8)
  line L14 (-8.85, 43.8) -> (-8.85, 42)
  line L15 (-8.85, 42) -> (-18.85, 42)
  line L16 (-18.85, 42) -> (-18.85, 6.5)
  line L17 (-18.85, 6.5) -> (-10.85, 6.5)
  line L18 (-10.85, 6.5) -> (-8.85, 4.5)
  line L19 (-8.85, 4.5) -> (-8.85, 0)
  line L20 (9.1614, 42) -> (18.1614, 42)
  line L21 (9.1614, 42) -> (9.1614, 22)
  line L22 (18.1614, 22) -> (9.1614, 22)
  line L23 (18.1614, 22) -> (18.1614, 42)
  line L24 (17.1614, 23) -> (17.1614, 41)
  line L25 (10.1614, 41) -> (17.1614, 41)
  line L26 (10.1614, 41) -> (10.1614, 23)
  line L27 (17.1614, 23) -> (10.1614, 23)
  line L28 (8.1614, 32) -> (10.1614, 32)
  line L29 (10.1614, 32) -> (10.1614, 34)
  line L30 (9.1614, 34) -> (10.1614, 34)
  line L31 (10.1614, 32) -> (10.1614, 30)
  line L32 (10.1614, 30) -> (9.1614, 30)
  line L33 (12, 38) -> (12.5, 38)
  line L34 (12.5, 38) -> (12.5, 37.5)
  line L35 (12.5, 37.5) -> (12, 37.5)
  line L36 (12, 37.5) -> (12, 38)
  line L37 (15, 38) -> (15.5, 38)
  line L38 (15, 37.5) -> (15, 38)
  line L39 (15.5, 38) -> (15.5, 37.5)
  line L40 (15.5, 37.5) -> (15, 37.5)
  line L41 (12, 35.25) -> (12.5, 35.25)
  line L42 (12, 34.75) -> (12, 35.25)
  line L43 (12.5, 35.25) -> (12.5, 34.75)
  line L44 (12.5, 34.75) -> (12, 34.75)
  line L45 (15, 35.25) -> (15.5, 35.25)
  line L46 (15, 34.75) -> (15, 35.25)
  line L47 (15.5, 35.25) -> (15.5, 34.75)
  line L48 (15.5, 34.75) -> (15, 34.75)
  line L49 (12, 32.5) -> (12.5, 32.5)
  line L50 (12, 32) -> (12, 32.5)
  line L51 (12.5, 32.5) -> (12.5, 32)
  line L52 (12.5, 32) -> (12, 32)
  line L53 (15, 32.5) -> (15.5, 32.5)
  line L54 (15, 32) -> (15, 32.5)
  line L55 (15.5, 32.5) -> (15.5, 32)
  line L56 (15.5, 32) -> (15, 32)
  line L57 (12, 29.75) -> (12.5, 29.75)
  line L58 (12, 29.25) -> (12, 29.75)
  line L59 (12.5, 29.75) -> (12.5, 29.25)
  line L60 (12.5, 29.25) -> (12, 29.25)
  line L61 (15, 29.75) -> (15.5, 29.75)
  line L62 (15, 29.25) -> (15, 29.75)
  line L63 (15.5, 29.75) -> (15.5, 29.25)
  line L64 (15.5, 29.25) -> (15, 29.25)
  line L65 (12, 27) -> (12.5, 27)
  line L66 (12, 26.5) -> (12, 27)
  line L67 (12.5, 27) -> (12.5, 26.5)
  line L68 (12.5, 26.5) -> (12, 26.5)
  line L69 (15, 27) -> (15.5, 27)
  line L70 (15, 26.5) -> (15, 27)
  line L71 (15.5, 27) -> (15.5, 26.5)
  line L72 (15.5, 26.5) -> (15, 26.5)
  dimension "d72" = 9
  dimension "d73" = 20
  dimension "d74" = 1
  dimension "d75" = 2
  dimension "d76" = 2
  dimension "d77" = 0.5
  dimension "d78" = 0.5
  dimension "d81" = 3
  dimension "d82" = -11
  constraint coincident L9 L20.start
  constraint perpendicular L9 L21
  constraint perpendicular L21 L22
  constraint perpendicular L9 L23
  constraint perpendicular L8 L28
  constraint midpoint L21 L28
  constraint perpendicular L28 L29
  constraint coincident L21 L30.start
  constraint perpendicular L26 L30
  constraint perpendicular L28 L31
  constraint coincident L21 L32.end
  constraint perpendicular L21 L32
  constraint horizontal L33
  constraint vertical L34
  constraint horizontal L35
  constraint vertical L36
  measures "d72" distance of L20.start L20.end
  measures "d73" distance of L20.start L21.end
  measures "d75" distance of L28.end L29.end
  measures "d76" distance of L28.end L31.end
  measures "d77" distance of L33.start L33.end
  measures "d78" distance of L33.start L35.end
extrude "Extrude8" add sketch "Sketch8" along normal blind 3 contours L9 L20 L21 L22 L23 L24 L25 L26 L27 L30 L32 | L21 L26 L28 L29 L30 | L21 L26 L28 L31 L32 | L24 L25 L26 L27 L29 L31
extrude "Extrude9" add sketch "Sketch8" along normal blind 13 contours L9 L20 L21 L22 L23 L24 L25 L26 L27 L30 L32
extrude "Extrude10" add sketch "Sketch8" along normal blind 9 contours L33 L34 L35 L36 | L37 L38 L39 L40 | L41 L42 L43 L44 | L45 L46 L47 L48 | L49 L50 L51 L52 | L53 L54 L55 L56 | L57 L58 L59 L60 | L61 L62 L63 L64 | L65 L66 L67 L68 | L69 L70 L71 L72
chamfer "Chamfer2" distance 0.2 angle 45 10 faces at (10.5, 12.1667, 37.8333) (10.5, 15.1667, 37.8333) (10.5, 12.1667, 35.0833) (10.5, 15.1667, 35.0833) (10.5, 12.1667, 32.3333) (10.5, 15.1667, 32.3333) (10.5, 15.1667, 29.5833) (10.5, 12.1667, 29.5833) (10.5, 15.1667, 26.8333) (10.5, 12.1667, 26.8333)
sketch "Sketch9" plane through (1.5, 0, 0) normal (1, 0, 0) x (0, 1, 0)
  line L0 (18.1614, 42) -> (18.1614, 22)
  line L1 (18.1614, 22) -> (9.1614, 22)
  line L2 (9.1614, 22) -> (9.1614, 42)
  line L3 (9.1614, 42) -> (8.85, 42)
  line L4 (8.85, 42) -> (8.85, 43.8)
  line L5 (8.85, 43.8) -> (2.5, 47.7)
  line L6 (2.5, 47.7) -> (-2.5, 47.7)
  line L7 (-2.5, 47.7) -> (-8.85, 43.8)
  line L8 (-8.85, 43.8) -> (-8.85, 42)
  line L9 (-8.85, 42) -> (-18.85, 42)
  line L10 (-18.85, 42) -> (-18.85, 6.5)
  line L11 (-18.85, 6.5) -> (-10.85, 6.5)
  line L12 (-10.85, 6.5) -> (-8.85, 4.5)
  line L13 (-8.85, 4.5) -> (-8.85, 0)
  line L14 (-8.85, 0) -> (8.85, 0)
  line L15 (8.85, 0) -> (8.85, 4.5)
  line L16 (8.85, 4.5) -> (10.85, 6.5)
  line L17 (10.85, 6.5) -> (18.85, 6.5)
  line L18 (18.85, 6.5) -> (18.85, 42)
  line L19 (18.85, 42) -> (18.1614, 42)
  line L20 (11.1, 13.4) -> (11.1, 20.9)
  line L21 (11.1, 20.9) -> (16.1, 20.9)
  line L22 (16.1, 20.9) -> (16.1, 13.4)
  line L23 (16.1, 13.4) -> (11.1, 13.4)
  line L24 (-18.85, 42) -> (-18.85, 27)
  line L25 (-18.85, 27) -> (-18.85, 34.3)
  line L26 (-18.85, 34.3) -> (-13.55, 34.3)
  line L27 (-13.55, 34.3) -> (-13.55, 27)
  line L28 (-13.55, 27) -> (-18.85, 27)
  line L29 (-17.5, 41.1) -> (-10.3, 41.1)
  line L30 (-17.5, 41.1) -> (-17.5, 37.1)
  line L31 (-17.5, 37.1) -> (-10.3, 37.1)
  line L32 (-10.3, 37.1) -> (-10.3, 41.1)
  line L33 (-14, 42) -> (-14, 41.1)
  circle A0 centre (1.55, 13.5) radius 3.2
  line L34 (1.55, 10.3) -> (1.55, 0)
  dimension "d90" = 15
  dimension "d91" = 7.3
  dimension "d92" = 5.3
  dimension "d93" = 7.2
  dimension "d94" = 4
  dimension "d95" = 0.9
  dimension "d98" = 6.4
  dimension "d119" = 10.3
  constraint coincident L9.end L10.start
  constraint perpendicular L9 L24
  constraint parallel L10 L25
  constraint perpendicular L24 L26
  constraint perpendicular L26 L27
  constraint perpendicular L10 L28
  constraint perpendicular L10 L29
  constraint perpendicular L29 L30
  constraint perpendicular L24 L31
  constraint perpendicular L29 L32
  constraint coincident L9 L33.start
  constraint coincident L29 L33.end
  constraint perpendicular L29 L33
  constraint coincident L14 L34.end
  constraint coincident A0 L34.start
  constraint perpendicular L14 L34
  measures "d90" distance of L9.end L24.end
  measures "d91" distance of L24.end L25.end
  measures "d92" distance of L25.end L26.end
  measures "d93" distance of L29.start L29.end
  measures "d94" distance of L29.start L30.end
  measures "d95" distance of L33.start L33.end
  measures "d98" diameter of A0
  measures "d119" distance of L34.end L34.start
extrude "Extrude11" add sketch "Sketch9" along normal blind 7.8 contours A0
fillet "Fillet1" radius 0.25 1 edges at (9.3, -1.4334, 12.3428)
extrude "Extrude12" add sketch "Sketch9" along normal blind 3 contours L10 L24 L25 L26 L27 L28
extrude "Extrude13" add sketch "Sketch9" along normal blind 7 contours L29 L30 L31 L32